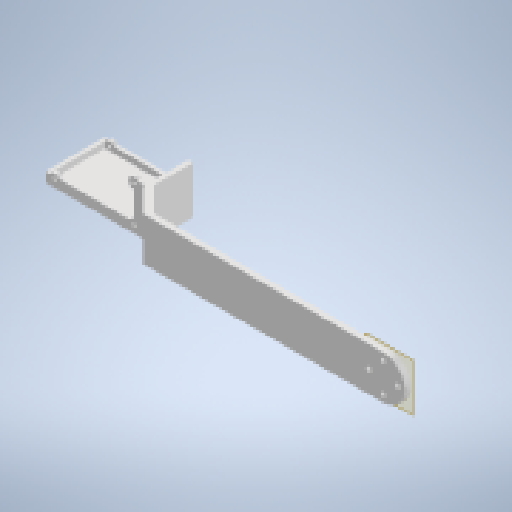
# Autodesk Inventor part: femurAux
Saved by Autodesk Inventor 2024 (Build 280153000, 153)
## iProperties
Created: 2024-03-17
Part Number: femurAux
Material: Genérico
Document SubType Name: Modeling
Designer: na_re
Density: 1 g/cm^3
Appearance: Valor por defecto
Author: na_re
Autodesk Inventor part; units mm, degrees
ref_plane "YZ Plane" through (0, 0, 0) normal (1, 0, 0) x (0, 1, 0)
ref_plane "XZ Plane" through (0, 0, 0) normal (0, 1, 0) x (-1, 0, 0)
ref_plane "XY Plane" through (0, 0, 0) normal (0, 0, 1) x (1, 0, 0)
ref_plane "Plano de trabajo1" through (0, 0, 0) normal (0, 0, 1) x (1, 0, 0)
sketch "Boceto1" plane through (0, 0, 0) normal (0, 0, 1) x (1, 0, 0)
  circle A0 centre (10.9923, -7.35) radius 1.2028 projected
  circle A1 centre (3.6423, 0) radius 1.2028 projected
  circle A2 centre (18.3423, 0) radius 1.2028 projected
  circle A3 centre (10.9923, 7.35) radius 1.2028 projected
  circle A4 centre (10.9923, 0) radius 10.9823 projected
  line L0 (10.9923, -10.9823) -> (-139.0077, -10.9823)
  line L1 (10.9923, 10.9823) -> (-139.0077, 10.9823)
  line L2 (-139.0077, 10.9823) -> (-139.0077, -10.9823)
  point P0 (0, 0)
  dimension "d0" = 150
  dimension "d1" = 150
  constraints: 6 end point, 2 horizontal, 2 point on circle, 1 perpendicular, 1 tangent
  measures "d0" distance of L0.start L0.end
  measures "d1" distance of L1.start L1.end
extrude "Extrusión1" add sketch "Boceto1" along normal blind 3
sketch "Boceto2" plane through (0, 0, 3) normal (0, 0, 1) x (1, 0, 0)
  arc A0 (-129.1978, -5.6745) -> (-132.1454, -8.5217) centre (-128.1245, -9.7351) ccw
  circle A1 centre (-128.1245, 8.4649) radius 0.85 construction
  circle A2 centre (-128.1245, -9.7351) radius 0.7049 construction
  line L0 (-139.0305, -11.0697) -> (-267.2186, 10.8953)
  line L1 (-267.2186, -11.0694) -> (-117.2186, -11.0694)
  line L2 (-139.0305, 10.8953) -> (-139.0305, -11.0694)
  line L3 (-117.2186, 10.8953) -> (-267.2186, 10.8953)
  line L4 (-128.1245, -11.0697) -> (-128.1245, -0.0872)
  line L5 (-128.1245, -0.0872) -> (-128.1245, 9.0128)
  line L6 (-128.1245, -0.0872) -> (-128.1245, -9.1872)
  circle A3 centre (-128.1245, -9.1872) radius 0.85
  circle A4 centre (-128.1245, 9.0128) radius 0.85
  circle A5 centre (-128.1245, -9.1872) radius 1.8825
  circle A6 centre (-128.1245, 9.0128) radius 1.8821
  circle A7 centre (-128.1245, 9.0128) radius 0.85
  circle A8 centre (-128.1245, -9.1872) radius 0.85
  line L7 (-128.1245, 10.8953) -> (-139.0305, 10.8953)
  line L8 (-139.0077, 10.9823) -> (-139.0077, -10.9823) projected
  line L9 (-139.0077, -10.9823) -> (-139.0077, 10.9823)
  line L10 (-139.0077, 10.9823) -> (-139.0077, -10.9823)
  point P0 (0, 0)
  dimension "d4" = 10.9825
  dimension "d5" = 9.1
  dimension "d6" = 9.1
  dimension "d7" = 1.7
  dimension "d8" = 1.7
  constraints: 20 end point, 8 centre point, 6 coincident, 3 point on line, 2 concentric, 2 point on circle, 1 parallel, 1 perpendicular, 1 vertical, 1 vertical alignment, 2 other
  measures "d4" distance of L4.start L5.start
  measures "d5" distance of L5.start L5.end
  measures "d6" distance of L5.start L6.end
  measures "d7" diameter of A3
  measures "d8" diameter of A4
extrude "Extrusión2" cut sketch "Boceto2" against normal blind 3 contours A3 L4 | L4 A3 | A4
sketch "Boceto3" plane through (0, 0, 3) normal (0, 0, 1) x (1, 0, 0)
  circle A0 centre (-128.1245, -9.1872) radius 0.85 projected
  circle A1 centre (-128.1245, 9.0128) radius 0.85 projected
  line L0 (10.9923, 10.9823) -> (-139.0077, 10.9823) projected
  line L1 (-139.0077, 10.9823) -> (-139.0077, -10.9823) projected
  line L2 (-139.0077, -10.9823) -> (10.9923, -10.9823) projected
  arc A2 (10.9923, -10.9823) -> (10.9923, 10.9823) centre (10.9923, 0) ccw projected
  circle A3 centre (10.9923, -7.35) radius 1.2028 projected
  circle A4 centre (3.6423, 0) radius 1.2028 projected
  circle A5 centre (18.3423, 0) radius 1.2028 projected
  circle A6 centre (10.9923, 7.35) radius 1.2028 projected
  line L3 (-130.1442, 5.5225) -> (-129.5361, 14.2169) projected
  circle A7 centre (-128.1245, -9.1872) radius 1.7951
  circle A8 centre (-128.1245, 9.0128) radius 1.9695
  line L4 (-128.1245, -7.3921) -> (-128.1245, 7.0432)
  line L5 (-128.1245, -10.9823) -> (-128.1245, -18.0451)
  line L6 (-128.1245, -18.0451) -> (-142.6221, -18.554)
  line L7 (-142.6221, -18.554) -> (-141.7315, 12.8288)
  line L8 (-141.7315, 12.8288) -> (-128.1245, 12.4426)
  line L9 (-128.1245, 12.4426) -> (-128.1245, 10.9823)
  point P0 (0, 0)
  constraints: 12 end point, 4 point on circle, 4 point on line, 2 centre point, 2 coincident, 2 tangent, 1 perpendicular, 1 vertical
extrude "Extrusión3" cut sketch "Boceto3" against normal blind 3 contours A8 L3 L0 | L3 A8 L4 A7 L2 L1 L0
sketch "Boceto4" plane through (0, 0, 0) normal (0, 0, -1) x (-1, 0, 0)
  arc A0 (128.1245, 7.0432) -> (128.1245, 10.9823) centre (128.1245, 9.0128) ccw projected
  line L0 (-10.9923, 10.9823) -> (128.1245, 10.9823) projected
  arc A1 (-10.9923, 10.9823) -> (-10.9923, -10.9823) centre (-10.9923, 0) ccw projected
  line L1 (128.1245, -10.9823) -> (-10.9923, -10.9823) projected
  arc A2 (128.1245, -10.9823) -> (128.1245, -7.3921) centre (128.1245, -9.1872) ccw projected
  line L2 (128.1245, -7.3921) -> (128.1245, 7.0432) projected
  circle A3 centre (128.1245, -9.1872) radius 0.85 projected
  circle A4 centre (128.1245, 9.0128) radius 0.85 projected
  circle A5 centre (-10.9923, -7.35) radius 1.2028 projected
  circle A6 centre (-3.6423, 0) radius 1.2028 projected
  circle A7 centre (-18.3423, 0) radius 1.2028 projected
  circle A8 centre (-10.9923, 7.35) radius 1.2028 projected
  line L3 (108.1857, 10.9823) -> (108.1857, -10.9823)
  point P0 (0, 0)
  constraints: 2 end point, 2 point on line, 1 perpendicular
extrude "Extrusión4" add sketch "Boceto4" along normal blind 12 contours L2 A2 L1 L3 L0 A0
sketch "Boceto5" plane through (0, 0, 3) normal (0, 0, 1) x (1, 0, 0)
  line L0 (-108.1857, -10.9823) -> (-108.1857, 10.9823) projected
  circle A0 centre (10.9923, 7.35) radius 1.2028 projected
  circle A1 centre (18.3423, 0) radius 1.2028 projected
  circle A2 centre (3.6423, 0) radius 1.2028 projected
  circle A3 centre (10.9923, -7.35) radius 1.2028 projected
  arc A4 (-128.1245, 10.9823) -> (-128.1245, 7.0432) centre (-128.1245, 9.0128) ccw projected
  line L1 (-128.1245, 7.0432) -> (-128.1245, -7.3921) projected
  arc A5 (-128.1245, -7.3921) -> (-128.1245, -10.9823) centre (-128.1245, -9.1872) ccw projected
  line L2 (-128.1245, -10.9823) -> (10.9923, -10.9823) projected
  arc A6 (10.9923, -10.9823) -> (10.9923, 10.9823) centre (10.9923, 0) ccw projected
  line L3 (10.9923, 10.9823) -> (-128.1245, 10.9823) projected
  circle A7 centre (-128.1245, 9.0128) radius 0.85 projected
  circle A8 centre (-128.1245, -9.1872) radius 0.85 projected
  line L4 (-108.1857, 10.9823) -> (-111.1857, 10.9823)
  line L5 (-111.1857, 10.9823) -> (-111.1857, -10.9823)
  line L6 (-111.1857, -10.9823) -> (-108.1857, -10.9823)
  line L7 (-108.1857, -10.9823) -> (-108.1857, 10.9823)
  line L8 (10.9923, 10.9823) -> (-128.1245, 10.9823) projected
  line L9 (-122.3999, 10.9823) -> (-122.3999, -10.9823)
  point P0 (0, 0)
  dimension "d15" = 3
  constraints: 10 end point, 3 point on line, 2 parallel, 2 perpendicular, 1 horizontal
  measures "d15" distance of L6.end L5.end
extrude "Extrusión5" cut sketch "Boceto5" against normal blind 13 contours L2 A5 L1 A4 L3 L9
chamfer "Chaflán1" distance 12 angle 45 1 edges at (-122.3999, 0, 3)
chamfer "Chaflán2" distance 12 angle 45 1 edges at (-108.1857, 0, -12)
sketch "Boceto6" plane through (0, 0, -12) normal (0, 0, -1) x (-1, 0, 0)
  line L0 (126.0445, -11.1372) -> (126.0445, 10.9228)
  line L1 (120.1857, -10.9823) -> (120.1857, 10.9823) projected
  line L2 (120.1857, -10.9823) -> (128.1245, -10.9823) projected
  line L3 (120.1857, 10.9823) -> (122.6857, 10.9823)
  line L4 (122.6857, 10.9823) -> (122.6857, -10.9823)
  line L5 (122.6857, -10.9823) -> (120.1857, -10.9823)
  line L6 (120.1857, -10.9823) -> (120.1857, 10.9823)
  point P0 (0, 0)
  dimension "d24" = 2.5
  constraints: 10 end point, 2 parallel, 1 horizontal, 1 perpendicular, 1 point on line, 1 vertical, 2 other
  measures "d24" distance of L4.end L5.end
extrude "Extrusión6" add sketch "Boceto6" along normal blind 20
sketch "Boceto7" plane through (-128.1245, -10.9823, -10) normal (0, -1, 0) x (1, 0, 0)
  line L0 (19.9388, 10) -> (7.9388, -2) projected
  line L1 (19.9388, 10) -> (139.1168, 10) projected
  line L2 (139.1168, 10) -> (139.1168, 13) projected
  line L3 (17.7246, 13) -> (139.1168, 13) projected
  line L4 (5.7246, 1) -> (17.7246, 13) projected
  line L5 (5.7246, 1) -> (5.7246, 0) projected
  line L6 (5.7246, 0) -> (0, 0) projected
  line L7 (0, 0) -> (0, -2) projected
  line L8 (5.4388, -2) -> (0, -2) projected
  line L9 (5.4388, -2) -> (5.4388, -22) projected
  line L10 (7.9388, -22) -> (5.4388, -22) projected
  line L11 (7.9388, -2) -> (7.9388, -22) projected
  line L12 (7.9388, -2) -> (7.9388, -22) projected
  line L13 (5.4388, -22) -> (7.9388, -22)
  line L14 (7.9388, -22) -> (7.9388, -4)
  line L15 (7.9388, -4) -> (5.4388, -4)
  line L16 (5.4388, -4) -> (5.4388, -22)
  point P0 (128.1245, 10)
  point P1 (5.4388, -4)
  dimension "d27" = 18
  constraints: 8 end point, 2 parallel, 1 horizontal, 1 perpendicular, 1 point on line
  measures "d27" distance of L14.end L13.end
extrude "Extrusión7" add sketch "Boceto7" along normal blind 2 contours L11 L10 L9 L15
sketch "Boceto8" plane through (-122.6857, -10.9823, -12) normal (-1, 0, 0) x (0, 0, 1)
  line L0 (0, 21.9646) -> (0, 0) projected
  line L1 (0, 21.9646) -> (-20, 21.9646) projected
  line L2 (-20, 21.9646) -> (-20, -2) projected
  line L3 (-2, -2) -> (-20, -2) projected
  line L4 (-2, 0) -> (-2, -2) projected
  line L5 (0, 0) -> (-2, 0) projected
  line L6 (-20, 0) -> (-2, 0)
  point P0 (12, 10.9823)
  constraints: 2 end point, 1 collinear, 1 point on line
extrude "Extrusión8" add sketch "Boceto8" along normal blind 50 contours L4 L3 L2 L6
sketch "Boceto9" plane through (-120.1857, -12.9823, -14) normal (0, 0, 1) x (1, 0, 0)
  line L0 (-2.5, 2) -> (0, 2) projected
  line L1 (-2.5, 2) -> (-52.5, 2) projected
  line L2 (-52.5, 0) -> (-52.5, 2) projected
  line L3 (0, 0) -> (-52.5, 0) projected
  line L4 (0, 2) -> (0, 0) projected
  line L5 (-2.5, 0) -> (-52.5, 0)
  line L6 (-52.5, 0) -> (-52.5, 2)
  line L7 (-52.5, 2) -> (-2.5, 2)
  line L8 (-2.5, 2) -> (-2.5, 0)
  point P0 (120.1857, 12.9823)
  constraints: 8 end point, 2 parallel, 1 horizontal, 1 perpendicular, 1 point on line
extrude "Extrusión9" add sketch "Boceto9" along normal blind 4 contours L8 L3 L2 L1
sketch "Boceto10" plane through (0, 0, -32) normal (0, 0, -1) x (-1, 0, 0)
  line L0 (120.1857, 10.9823) -> (120.1857, -12.9823) projected
  line L1 (120.1857, -12.9823) -> (172.6857, -12.9823) projected
  line L2 (172.6857, -10.9823) -> (172.6857, -12.9823) projected
  line L3 (122.6857, -10.9823) -> (172.6857, -10.9823) projected
  line L4 (122.6857, 10.9823) -> (122.6857, -10.9823) projected
  line L5 (122.6857, 10.9823) -> (120.1857, 10.9823) projected
  line L6 (133.3495, -12.9823) -> (133.3495, -10.9823)
  line L7 (128.1245, -10.9823) -> (172.6857, -10.9823) projected
  point P0 (0, 0)
  constraints: 2 end point, 2 point on line, 1 perpendicular
extrude "Extrusión10" add sketch "Boceto10" along normal blind 8 contours L6 L3 L2 L1
sketch "Boceto11" plane through (-172.6857, -10.9823, -10) normal (0, 1, 0) x (1, 0, 0)
  line L0 (50, 22) -> (50, 4) projected
  line L1 (50, 22) -> (39.3362, 22) projected
  line L2 (39.3362, 22) -> (39.3362, 30) projected
  line L3 (0, 30) -> (39.3362, 30) projected
  line L4 (0, 30) -> (0, 0) projected
  line L5 (44.5612, 0) -> (0, 0) projected
  line L6 (44.5612, 0) -> (44.5612, 2) projected
  line L7 (50, 2) -> (44.5612, 2) projected
  line L8 (50, 2) -> (50, 4) projected
  line L9 (39.3362, 22) -> (39.3362, 30) projected
  line L10 (39.3362, 30) -> (39.3362, 28)
  line L11 (39.3362, 28) -> (0, 28)
  line L12 (0, 28) -> (2, 28)
  line L13 (2, 28) -> (2, 0)
  line L14 (0, 0) -> (0, 30) projected
  line L15 (0, 0) -> (0, 2)
  line L16 (0, 2) -> (43.0714, 2)
  line L17 (43.0714, 2) -> (43.0714, 0)
  line L18 (44.5612, 0) -> (0, 0) projected
  point P0 (172.6857, -10)
  point P1 (2, 2)
  point P2 (39.3362, 28)
  dimension "d36" = 2
  dimension "d37" = 2
  dimension "d38" = 2
  constraints: 14 end point, 7 point on line, 3 perpendicular
  measures "d36" distance of L2.end L10.end
  measures "d37" distance of L11.end L12.end
  measures "d38" distance of L4.end L15.end
extrude "Extrusión11" add sketch "Boceto11" along normal blind 3 contours L11 L4 L3 L2 | L13 L16 L4 L11 | L16 L17 L5 L13 | L13 L5 L4 L16
sketch "Boceto12" plane through (0, 0, -40) normal (0, 0, -1) x (-1, 0, 0)
  circle A0 centre (168.3345, -9.2072) radius 0.85
  point P0 (0, 0)
  constraints: 1 centre point, 2 other
extrude "Extrusión12" cut sketch "Boceto12" against normal blind 35
sketch "Boceto13" plane through (0, 0, -12) normal (0, 0, -1) x (-1, 0, 0)
  circle A0 centre (168.3345, -9.2072) radius 0.85 projected
  circle A1 centre (128.1245, 9.0128) radius 0.85 projected
  circle A2 centre (128.1245, -9.1872) radius 0.85 projected
  arc A3 (129.6143, -8.1857) -> (128.1245, -7.3921) centre (128.1245, -9.1872) ccw projected
  line L0 (128.1245, -7.3921) -> (128.1245, 7.0432) projected
  arc A4 (128.1245, 7.0432) -> (128.1245, 10.9823) centre (128.1245, 9.0128) ccw projected
  line L1 (128.1245, 10.9823) -> (122.6857, 10.9823) projected
  line L2 (122.6857, 10.9823) -> (122.6857, -10.9823) projected
  line L3 (122.6857, -10.9823) -> (128.1245, -10.9823) projected
  arc A5 (128.1245, -10.9823) -> (129.6143, -10.1887) centre (128.1245, -9.1872) ccw projected
  line L4 (129.6143, -10.9823) -> (129.6143, -10.1887) projected
  line L5 (170.6857, -10.9823) -> (129.6143, -10.9823) projected
  line L6 (170.6857, -10.9823) -> (170.6857, -7.9823) projected
  line L7 (129.6143, -7.9823) -> (170.6857, -7.9823) projected
  line L8 (129.6143, -8.1857) -> (129.6143, -7.9823) projected
  circle A6 centre (128.1245, 9.0128) radius 2.7195
  circle A7 centre (128.1245, -9.1872) radius 2.545
  point P0 (0, 0)
  point P1 (126.3205, -10.9823)
  point P2 (129.9286, -10.9823)
  point P3 (130.3662, -7.9823)
  point P4 (128.1245, -6.6422)
  point P5 (128.1245, 6.2933)
  point P6 (126.2493, 10.9823)
  dimension "d43" = 5.439
  dimension "d44" = 5.09
  constraints: 2 centre point, 2 coincident
  measures "d43" diameter of A6
  measures "d44" diameter of A7
extrude "Extrusión13" add sketch "Boceto13" against normal blind 2 contours A3 L0 A7 L7 L8 | L0 A4 L1 A6 | L3 A5 L4 L5 A7 picked at (127.0429, 11.109)
sketch "Boceto14" plane through (0, 0, -10) normal (0, 0, 1) x (1, 0, 0)
  circle A0 centre (-128.1245, -9.1872) radius 0.85 projected
  arc A1 (-128.1245, -6.6422) -> (-130.3662, -7.9823) centre (-128.1245, -9.1872) ccw projected
  circle A2 centre (-168.3345, -9.2072) radius 0.85 projected
  circle A3 centre (-168.3345, -9.2072) radius 0.85 projected
  circle A4 centre (-168.3345, -9.2072) radius 2.545
  line L0 (-172.6857, -7.9823) -> (-130.3662, -7.9823) projected
  point P0 (0, 0)
  point P1 (-170.5654, -7.9823)
  point P2 (-166.1037, -7.9823)
  dimension "d47" = 5.09
  constraints: 1 centre point, 1 coincident
  measures "d47" diameter of A4
extrude "Extrusión14" add sketch "Boceto14" against normal blind 2 contours L0 A4 picked at (-168.0387, -7.2686)
sketch "Boceto15" plane through (0, 0, -40) normal (0, 0, -1) x (-1, 0, 0)
  circle A0 centre (168.3345, -9.2072) radius 0.85 projected
  circle A1 centre (168.3345, -9.2072) radius 2.545
  line L0 (133.3495, -7.9823) -> (172.6857, -7.9823) projected
  point P0 (0, 0)
  point P1 (166.1037, -7.9823)
  point P2 (170.5654, -7.9823)
  dimension "d50" = 5.09
  constraints: 1 centre point, 1 coincident
  measures "d50" diameter of A1
extrude "Extrusión15" add sketch "Boceto15" against normal blind 2 contours L0 A1 picked at (168.6303, -7.2686)
